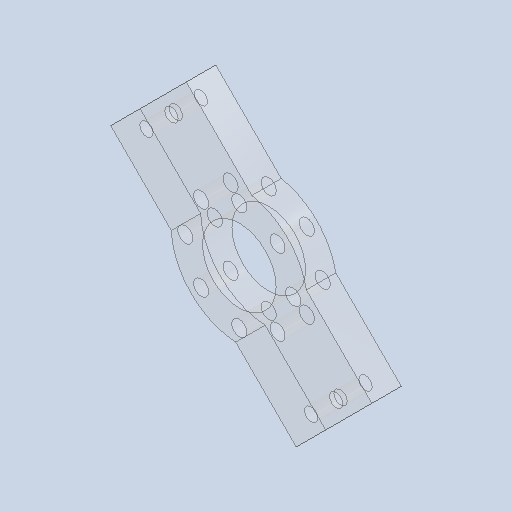
# Autodesk Inventor part: _arm_pti
Saved by Autodesk Inventor 2024.3 (Build 283343000, 343)
## iProperties
Created: 2024-09-09
Part Number: _arm_pti
Material: PMMA 플라스틱
Document SubType Name: Modeling
Designer: gretc
Density: 1.188 g/cm^3
Appearance: 폴리카보네이트 - 선명
Mass: 6.9695 g
Surface Area: 38.2948 cm^2
Volume: 5.86658 cm^3
Author: gretc
Autodesk Inventor part; units mm, degrees
ref_plane "YZ Plane" through (0, 0, 0) normal (1, 0, 0) x (0, 1, 0)
ref_plane "XZ Plane" through (0, 0, 0) normal (0, 1, 0) x (-1, 0, 0)
ref_plane "XY Plane" through (0, 0, 0) normal (0, 0, 1) x (1, 0, 0)
sketch "스케치1" plane through (0, 0, 0) normal (0, 0, 1) x (1, 0, 0)
  circle A0 centre (-7.7782, -7.7782) radius 1.55 projected
  circle A1 centre (7.7782, -7.7782) radius 1.55 projected
  circle A2 centre (7.7782, 7.7782) radius 1.55 projected
  circle A3 centre (-7.7782, 7.7782) radius 1.55 projected
  circle A4 centre (0, 0) radius 5 projected
  circle A5 centre (0, 0) radius 13.9 projected
  circle A6 centre (0, 11) radius 1.55 projected
  circle A7 centre (11, 0) radius 1.55 projected
  circle A8 centre (0, -11) radius 1.55 projected
  circle A9 centre (-11, 0) radius 1.55 projected
  line L0 (27.0238, -10.8065) -> (11.6088, -26.2214) projected
  line L1 (-10.8065, 27.0238) -> (-26.2214, 11.6088) projected
  line L2 (-10.8065, 27.0238) -> (-26.2214, 11.6088) projected
  line L3 (-10.8065, 27.0238) -> (-26.2214, 11.6088)
  line L4 (-26.2214, 11.6088) -> (11.6088, -26.2214)
  line L5 (11.6088, -26.2214) -> (27.0238, -10.8065)
  line L6 (27.0238, -10.8065) -> (-10.8065, 27.0238)
  line L7 (11.6795, -26.1507) -> (26.9531, -10.8772) projected
  line L8 (26.9531, -10.8772) -> (22.7104, -6.6345) projected
  line L9 (7.4369, -21.908) -> (22.7104, -6.6345) projected
  line L10 (11.6795, -26.1507) -> (7.4369, -21.908) projected
  circle A10 centre (0, 0) radius 7.5 projected
  point P0 (0, 0)
  point P1 (-13.8807, -0.7318)
  point P2 (-0.7318, -13.8807)
  point P3 (13.6634, 2.554)
  point P4 (2.554, 13.6634)
  constraints: 8 end point, 3 equal length, 1 perpendicular
extrude "돌출1" add sketch "스케치1" along normal blind 6 contours A0 L4 A5 L6 A2 | A0 L4 A5 | L4 L1 L6 A5 | A5 L6 L0 L8 L9 L10 L4 | A5 L6 A2 | L10 L9 L8 L0
sketch "스케치2" plane through (0, 0, 0) normal (0, 0, -1) x (-1, 0, 0)
  circle A0 centre (13.847, 19.7406) radius 1.35 projected
  circle A1 centre (18.9382, 14.6494) radius 1.35 projected
  circle A2 centre (-14.6494, -18.9382) radius 1.35 projected
  circle A3 centre (-19.7406, -13.847) radius 1.35 projected
  point P0 (0, 0)
extrude "돌출2" cut sketch "스케치2" against normal blind 6
